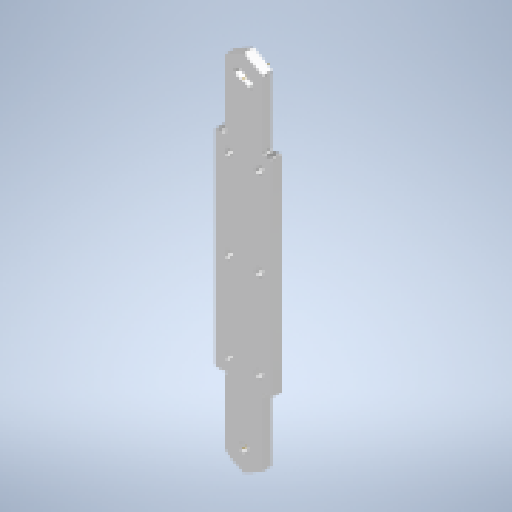
# Autodesk Inventor part: Z-Axis Nut and Bed Plate RevIII
Saved by Autodesk Inventor 2024 (Build 280153000, 153)
## iProperties
Created: 2024-08-02
Part Number: Z-Axis Nut and Bed Plate RevIII
Material: Aluminum 6061
Document SubType Name: Modeling
Designer: Ishaan
Density: 2.7 g/cm^3
Appearance: Aluminum - Flat
Author: Ishaan
Autodesk Inventor part; units mm, degrees
ref_plane "YZ Plane" through (0, 0, 0) normal (1, 0, 0) x (0, 1, 0)
ref_plane "XZ Plane" through (0, 0, 0) normal (0, 1, 0) x (-1, 0, 0)
ref_plane "XY Plane" through (0, 0, 0) normal (0, 0, 1) x (1, 0, 0)
sketch "Sketch1" plane through (0, 0, 0) normal (0, 0, 1) x (1, 0, 0)
  line L0 (12.5, -112.2169) -> (-12.5, -112.2169)
  line L1 (-12.5, -112.2169) -> (-12.5, 112.2169)
  line L2 (-12.5, 112.2169) -> (12.5, 112.2169)
  line L3 (12.5, 112.2169) -> (12.5, -112.2169)
  line L4 (12.5, -112.2169) -> (-12.5, 112.2169) construction
  line L5 (-12.5, -112.2169) -> (12.5, 112.2169) construction
  line L6 (0, 105) -> (0, -105) construction
  line L7 (-12.5, 112.2169) -> (0, 119.4338)
  line L8 (0, 119.4338) -> (12.5, 112.2169)
  line L9 (12.5, 112.2169) -> (12.5, 97.7831)
  line L10 (12.5, 97.7831) -> (0, 90.5662)
  line L11 (0, 90.5662) -> (-12.5, 97.7831)
  line L12 (-12.5, 97.7831) -> (-12.5, 112.2169)
  line L13 (-12.5, -112.2169) -> (-12.5, -97.7831)
  line L14 (-12.5, -97.7831) -> (0, -90.5662)
  line L15 (0, -90.5662) -> (12.5, -97.7831)
  line L16 (12.5, -97.7831) -> (12.5, -112.2169)
  line L17 (12.5, -112.2169) -> (0, -119.4338)
  line L18 (0, -119.4338) -> (-12.5, -112.2169)
  line L19 (-4.1551, 106.7278) -> (4.1551, 103.2722) construction
  line L20 (-4.9806, 104.7427) -> (3.3295, 101.287)
  line L21 (4.9806, 105.2573) -> (-3.3295, 108.713)
  arc A0 (-3.3295, 108.713) -> (-4.9806, 104.7427) centre (-4.1551, 106.7278) ccw
  arc A1 (3.3295, 101.287) -> (4.9806, 105.2573) centre (4.1551, 103.2722) ccw
  circle A2 centre (0, -105) radius 3.5
  line L22 (18.5, -67.75) -> (-18.5, -67.75)
  line L23 (-18.5, -67.75) -> (-18.5, 67.75)
  line L24 (-18.5, 67.75) -> (18.5, 67.75)
  line L25 (18.5, 67.75) -> (18.5, -67.75)
  line L26 (18.5, -67.75) -> (-18.5, 67.75) construction
  line L27 (-18.5, -67.75) -> (18.5, 67.75) construction
  circle A3 centre (0, 0) radius 12.7
  point P0 (252.5, 0)
  point P1 (-12.5, -67.75)
  point P2 (12.5, -112.2169)
  point P3 (-12.5, 67.75)
  point P4 (12.5, 67.75)
  point P5 (12.5, -67.75)
  point P6 (12.5, 97.7831)
  point P7 (-12.5, 112.2169)
  point P8 (12.5, -97.7831)
  point P9 (-12.5, -112.2169)
  point P10 (12.5, -112.2169)
  point P11 (12.5, -2.245)
  point P12 (-12.5, -2.245)
  point P13 (-12.5, 2.245)
  point P14 (12.5, 2.245)
  dimension "d0" = 25
  dimension "d1" = 252.5
  dimension "d2" = 210
  dimension "d3" = 4.3
  dimension "d4" = 9
  dimension "d5" = 7
  dimension "d12" = 135.5
  dimension "d13" = 37
  dimension "d43" = 25.4
  constraints: 58 end point, 6 midpoint, 5 parallel, 4 centre point, 4 coincident, 4 point on circle, 4 tangent, 2 collinear, 2 horizontal, 2 perpendicular, 2 point on line, 1 horizontal alignment, 1 vertical, 26 other
  measures "d0" distance of L2.end L1.end
  measures "d1" distance of point (252.5, 0) point (0, 0)
  measures "d2" distance of L6.start L6.end
  measures "d3" diameter of A1
  measures "d4" distance of L19.start L19.end
  measures "d5" diameter of A2
  measures "d12" distance of L24.end L22.start
  measures "d13" distance between parallel lines of L25 L23
  measures "d43" diameter of A3
extrude "Extrusion1" add sketch "Sketch1" along normal blind 6.35
sketch "Sketch2" plane through (0, 0, 6.35) normal (0, 0, 1) x (1, 0, 0)
  line L0 (-18.5, 67.75) -> (-18.5, -67.75) projected
  line L1 (-18.5, -67.75) -> (-12.5, -67.75) projected
  line L2 (-12.5, -67.75) -> (-12.5, -112.2169) projected
  line L3 (-12.5, -112.2169) -> (0, -119.4338) projected
  line L4 (0, -119.4338) -> (12.5, -112.2169) projected
  line L5 (12.5, -112.2169) -> (12.5, -67.75) projected
  line L6 (12.5, -67.75) -> (18.5, -67.75) projected
  line L7 (18.5, -67.75) -> (18.5, 67.75) projected
  line L8 (18.5, 67.75) -> (12.5, 67.75) projected
  line L9 (12.5, 67.75) -> (12.5, 112.2169) projected
  line L10 (12.5, 112.2169) -> (0, 119.4338) projected
  line L11 (0, 119.4338) -> (-12.5, 112.2169) projected
  line L12 (-12.5, 112.2169) -> (-12.5, 67.75) projected
  line L13 (-12.5, 67.75) -> (-18.5, 67.75) projected
  arc A0 (-3.3295, 108.713) -> (-4.9806, 104.7427) centre (-4.1551, 106.7278) ccw projected
  line L14 (-3.3295, 108.713) -> (4.9806, 105.2573) projected
  arc A1 (3.3295, 101.287) -> (4.9806, 105.2573) centre (4.1551, 103.2722) ccw projected
  line L15 (3.3295, 101.287) -> (-4.9806, 104.7427) projected
  circle A2 centre (0, -105) radius 3.5 projected
  circle A3 centre (-13.25, 68.5) radius 1.375
  point P0 (0, 0)
  point P1 (-12.5, 69.6524)
  point P2 (-14.4024, 67.75)
  dimension "d16" = 0.75
  dimension "d17" = 2.75
  dimension "d18" = 0.75
  constraints: 1 centre point
  measures "d16" distance from line of L12 A3.centre
  measures "d17" diameter of A3
  measures "d18" distance from line of A3.centre L13
extrude "Extrusion2" cut sketch "Sketch2" against normal through all contours L13 L12 A3 picked at (-12.4132, 68.945)
mirror "Mirror1" about plane through (0, 0, 0) normal (1, 0, 0) of "Extrusion2"
mirror "Mirror2" about plane through (0, 0, 0) normal (0, 1, 0) of "Extrusion2", "Mirror1"
sketch "Sketch4" plane through (0, 0, 6.35) normal (0, 0, 1) x (1, 0, 0)
  line L0 (-18.5, -67.75) -> (-14.4024, -67.75) construction
  line L1 (10, -58) -> (-10, -58) construction
  line L2 (-10, -58) -> (-10, 58) construction
  line L3 (-10, 58) -> (10, 58) construction
  line L4 (10, 58) -> (10, -58) construction
  line L5 (10, -58) -> (-10, 58) construction
  line L6 (-10, -58) -> (10, 58) construction
  point P0 (0, 0)
  point P1 (10, 0)
  point P2 (-10, 0)
  dimension "d45" = 20
  dimension "d46" = 116
  constraints: 12 end point, 4 coincident, 4 midpoint, 2 parallel, 1 horizontal, 1 perpendicular
  measures "d45" distance of L2.end L3.end
  measures "d46" distance of L1.end L2.end
hole "Hole2" at (10, -58, 6.35) at (-10, -58, 6.35) at (-10, 0, 6.35) at (10, 0, 6.35) at (10, 58, 6.35) at (-10, 58, 6.35) direction (0, 0, -1) diameter 5.3 end through all
fillet "Fillet3" radius 1 18 edges at (-18.5, 67.75, 3.175) (-18.5, -67.75, 3.175) (14.4024, -67.75, 3.175) (-14.4024, -67.75, 3.175) (-12.5, -69.6524, 3.175) (18.5, -67.75, 3.175) (12.5, -69.6524, 3.175) (0, -119.4338, 3.175) (12.5, -112.2169, 3.175) (-12.5, -112.2169, 3.175) (18.5, 67.75, 3.175) (-14.4024, 67.75, 3.175) (14.4024, 67.75, 3.175) (0, 119.4338, 3.175) (-12.5, 112.2169, 3.175) (-12.5, 69.6524, 3.175) (12.5, 69.6524, 3.175) (12.5, 112.2169, 3.175)
equation "\"d18\" = d16"
body "Solid1"
